Autodesk Fusion 360 part; units mm, degrees
(part 2 of 4)
sketch "Sketch14" plane through (0, 0, 0.5) normal (0, 0, 1) x (-1, 0, 0)
  circle A0 centre (101.6789, -8.3211) radius 5
  circle A1 centre (108.75, -80) radius 2
  circle A2 centre (86.25, -80) radius 2
  circle A3 centre (63.75, -80) radius 2
  circle A4 centre (41.25, -77.5) radius 2
  circle A5 centre (73.3947, -36.6053) radius 5
  circle A6 centre (87.5368, -22.4632) radius 5
  line L0 (120, -80) -> (120, 10)
  line L1 (120, 10) -> (75, 10)
  line L2 (75, 10) -> (30, 0)
  line L3 (30, 0) -> (0, 0)
  line L4 (0, 0) -> (-45, 10)
  line L5 (-45, 10) -> (-75.7574, 10)
  line L6 (-75.7574, 10) -> (-181.8234, 116.066)
  line L7 (-181.8234, 116.066) -> (-195.9655, 101.9239)
  line L8 (-195.9655, 101.9239) -> (-90, -4.0416)
  line L9 (-90, -4.0416) -> (-90, -62.2885)
  line L10 (-90, -62.2885) -> (-190, -62.2885)
  line L11 (-190, -62.2885) -> (-190, -75)
  line L12 (-190, -75) -> (-90, -75)
  line L13 (-90, -75) -> (-90, -80)
  line L14 (-90, -80) -> (-22.5, -80)
  line L15 (-22.5, -80) -> (0, -75)
  line L16 (0, -75) -> (30, -75)
  line L17 (30, -75) -> (37.3453, -76.6323)
  line L18 (37.3453, -76.6323) -> (37.3453, -83.3677)
  line L19 (37.3453, -83.3677) -> (45.1547, -83.3677)
  line L20 (45.1547, -83.3677) -> (45.1547, -78.3677)
  line L21 (45.1547, -78.3677) -> (52.5, -80)
  line L22 (52.5, -80) -> (59.75, -80)
  line L23 (59.75, -80) -> (59.75, -85)
  line L24 (59.75, -85) -> (67.75, -85)
  line L25 (67.75, -85) -> (67.75, -80)
  line L26 (67.75, -80) -> (82.25, -80)
  line L27 (82.25, -80) -> (82.25, -85)
  line L28 (82.25, -85) -> (90.25, -85)
  line L29 (90.25, -85) -> (90.25, -80)
  line L30 (90.25, -80) -> (104.75, -80)
  line L31 (104.75, -80) -> (104.75, -85)
  line L32 (104.75, -85) -> (112.75, -85)
  line L33 (112.75, -85) -> (112.75, -80)
  line L34 (112.75, -80) -> (120, -80)
  line L35 (-14.25, -68.5) -> (-8.25, -68.5)
  line L36 (-8.25, -68.5) -> (-8.25, -71.5)
  line L37 (-8.25, -71.5) -> (-14.25, -71.5)
  line L38 (-14.25, -71.5) -> (-14.25, -68.5)
  line L39 (-72.1594, -47.0213) -> (-67.271, -50.5004)
  line L40 (-67.271, -50.5004) -> (-69.0348, -52.9787)
  line L41 (-69.0348, -52.9787) -> (-73.9232, -49.4996)
  line L42 (-73.9232, -49.4996) -> (-72.1594, -47.0213)
  line L43 (-58.1594, -27.0213) -> (-53.271, -30.5004)
  line L44 (-53.271, -30.5004) -> (-55.0348, -32.9787)
  line L45 (-55.0348, -32.9787) -> (-59.9232, -29.4996)
  line L46 (-59.9232, -29.4996) -> (-58.1594, -27.0213)
  line L47 (-10.5728, -3.1023) -> (-4.573, -3.1532)
  line L48 (-4.573, -3.1532) -> (-4.5984, -6.1531)
  line L49 (-4.5984, -6.1531) -> (-10.5982, -6.1022)
  line L50 (-10.5982, -6.1022) -> (-10.5728, -3.1023)
  line L51 (-67.8203, 7.9003) -> (-65.8203, 7.9003)
  line L52 (-65.8203, 7.9003) -> (-65.8203, 5.9003)
  line L53 (-65.8203, 5.9003) -> (-67.8203, 5.9003)
  line L54 (-67.8203, 5.9003) -> (-67.8203, 7.9003)
  line L55 (-76.9306, -16.181) -> (-75.5164, -17.5952)
  line L56 (-75.5164, -17.5952) -> (-76.9306, -19.0095)
  line L57 (-76.9306, -19.0095) -> (-78.3448, -17.5952)
  line L58 (-78.3448, -17.5952) -> (-76.9306, -16.181)
  line L59 (-87.8309, -27.9541) -> (-85.8309, -27.9541)
  line L60 (-85.8309, -27.9541) -> (-85.8309, -29.9541)
  line L61 (-85.8309, -29.9541) -> (-87.8309, -29.9541)
  line L62 (-87.8309, -29.9541) -> (-87.8309, -27.9541)
  line L63 (-66.3319, -10.7541) -> (-65.4866, -8.9415)
  line L64 (-65.4866, -8.9415) -> (-63.674, -9.7867)
  line L65 (-63.674, -9.7867) -> (-64.5193, -11.5994)
  line L66 (-64.5193, -11.5994) -> (-66.3319, -10.7541)
  line L67 (-42.179, 1.1199) -> (-36.1792, 1.0739)
  line L68 (-36.1792, 1.0739) -> (-36.2025, -1.9678)
  line L69 (-36.2025, -1.9678) -> (-42.2023, -1.9219)
  line L70 (-42.2023, -1.9219) -> (-42.179, 1.1199)
  line L71 (-10.5728, -25.1023) -> (-4.573, -25.1532)
  line L72 (-4.573, -25.1532) -> (-4.5984, -28.1531)
  line L73 (-4.5984, -28.1531) -> (-10.5982, -28.1022)
  line L74 (-10.5982, -28.1022) -> (-10.5728, -25.1023)
  line L75 (-11.9719, -47.9791) -> (-6.0721, -49.071)
  line L76 (-6.0721, -49.071) -> (-6.6181, -52.0209)
  line L77 (-6.6181, -52.0209) -> (-12.5179, -50.929)
  line L78 (-12.5179, -50.929) -> (-11.9719, -47.9791)
  line L79 (-81.75, -71.5367) -> (-75.75, -71.5367)
  line L80 (-75.75, -71.5367) -> (-75.75, -74.5367)
  line L81 (-75.75, -74.5367) -> (-81.75, -74.5367)
  line L82 (-81.75, -74.5367) -> (-81.75, -71.5367)
  line L83 (-36.75, -71.5367) -> (-30.75, -71.5367)
  line L84 (-30.75, -71.5367) -> (-30.75, -74.5367)
  line L85 (-30.75, -74.5367) -> (-36.75, -74.5367)
  line L86 (-36.75, -74.5367) -> (-36.75, -71.5367)
  line L87 (-50.7607, -47.5524) -> (-45.1333, -49.6339)
  line L88 (-45.1333, -49.6339) -> (-46.174, -52.4476)
  line L89 (-46.174, -52.4476) -> (-51.8014, -50.3661)
  line L90 (-51.8014, -50.3661) -> (-50.7607, -47.5524)
  line L91 (-43.7607, -25.5524) -> (-38.1333, -27.6339)
  line L92 (-38.1333, -27.6339) -> (-39.174, -30.4476)
  line L93 (-39.174, -30.4476) -> (-44.8014, -28.3661)
  line L94 (-44.8014, -28.3661) -> (-43.7607, -25.5524)
  line L95 (-24.686, 0.859) -> (-18.6861, 0.8794)
  line L96 (-18.6861, 0.8794) -> (-18.6759, -2.1206)
  line L97 (-18.6759, -2.1206) -> (-24.6759, -2.141)
  line L98 (-24.6759, -2.141) -> (-24.686, 0.859)
  line L99 (-62.1634, 5.9003) -> (-62.1634, 7.9003)
  line L100 (-62.1634, 7.9003) -> (-60.1634, 7.9003)
  line L101 (-60.1634, 7.9003) -> (-60.1634, 5.9003)
  line L102 (-60.1634, 5.9003) -> (-62.1634, 5.9003)
  line L103 (-72.9306, -20.181) -> (-71.5164, -21.5952)
  line L104 (-71.5164, -21.5952) -> (-72.9306, -23.0095)
  line L105 (-72.9306, -23.0095) -> (-74.3448, -21.5952)
  line L106 (-74.3448, -21.5952) -> (-72.9306, -20.181)
  line L107 (-87.8309, -19.8881) -> (-85.8309, -19.8881)
  line L108 (-85.8309, -19.8881) -> (-85.8309, -21.8881)
  line L109 (-85.8309, -21.8881) -> (-87.8309, -21.8881)
  line L110 (-87.8309, -21.8881) -> (-87.8309, -19.8881)
  line L111 (-70.6135, -6.5508) -> (-68.8009, -7.396)
  line L112 (-68.8009, -7.396) -> (-69.6461, -9.2087)
  line L113 (-69.6461, -9.2087) -> (-71.4587, -8.3634)
  line L114 (-71.4587, -8.3634) -> (-70.6135, -6.5508)
  line L115 (-35.0324, 0.9507) -> (-29.0325, 0.9195)
  line L116 (-29.0325, 0.9195) -> (-29.0481, -2.0804)
  line L117 (-29.0481, -2.0804) -> (-35.048, -2.0492)
  line L118 (-35.048, -2.0492) -> (-35.0324, 0.9507)
  line L119 (-28.0908, -25.011) -> (-22.1784, -26.0328)
  line L120 (-22.1784, -26.0328) -> (-22.6893, -28.989)
  line L121 (-22.6893, -28.989) -> (-28.6017, -27.9672)
  line L122 (-28.6017, -27.9672) -> (-28.0908, -25.011)
  line L123 (-26.6893, -51.989) -> (-32.6017, -50.9672)
  line L124 (-32.6017, -50.9672) -> (-32.0908, -48.011)
  line L125 (-32.0908, -48.011) -> (-26.1784, -49.0328)
  line L126 (-26.1784, -49.0328) -> (-26.6893, -51.989)
  line L127 (-59.25, -71.5367) -> (-53.25, -71.5367)
  line L128 (-53.25, -71.5367) -> (-53.25, -74.5367)
  line L129 (-53.25, -74.5367) -> (-59.25, -74.5367)
  line L130 (-59.25, -74.5367) -> (-59.25, -71.5367)
  line L131 (-45, -57) -> (-5, -57)
  line L132 (-5, -57) -> (-5, -60)
  line L133 (-5, -60) -> (-45, -60)
  arc A7 (-45, -60) -> (-66.3234, -75) centre (-45, -82.6562) ccw
  line L134 (-66.3234, -75) -> (-69.4872, -75)
  arc A8 (-45, -57) -> (-69.4872, -75) centre (-45, -82.6562) ccw
  line L135 (0, -5) -> (30, -5)
  line L136 (30, -5) -> (30, -70)
  line L137 (30, -70) -> (0, -70)
  line L138 (0, -70) -> (0, -5)
  circle A9 centre (-167.6812, 87.7817) radius 5
  circle A10 centre (-120, -68.6442) radius 5
  circle A11 centre (-140, -68.6442) radius 5
  circle A12 centre (-153.5391, 73.6396) radius 5
  arc A13 (-87.8309, -44.505) -> (-40.6089, 7.444) centre (-128.4491, 39.8542) ccw
  line L139 (-87.8309, -44.505) -> (-87.8309, -38.9188)
  arc A14 (-87.8309, -38.9188) -> (-45.6219, 8.3158) centre (-128.4491, 39.8542) ccw
  line L140 (-45.6219, 8.3158) -> (-40.6089, 7.444)
  circle A15 centre (-181.8234, 101.9239) radius 5
  circle A16 centre (-160, -68.6442) radius 5
  circle A17 centre (-180, -68.6442) radius 5
  circle A18 centre (-139.397, 59.4975) radius 5
  circle A19 centre (-125.2548, 45.3553) radius 5
  circle A20 centre (-111.1127, 31.2132) radius 5
  line L141 (30, -70) -> (120, -70)
  line L142 (108.75, -85) -> (108.75, -59.5533)
  circle A21 centre (108.75, -70) radius 2
  circle A22 centre (105.25, -70) radius 1.5 construction
  circle A23 centre (101.75, -70) radius 2
  circle A24 centre (98.25, -70) radius 1.5 construction
  circle A25 centre (94.75, -70) radius 2
  circle A26 centre (91.25, -70) radius 1.5 construction
  circle A27 centre (87.75, -70) radius 2
  circle A28 centre (84.25, -70) radius 1.5 construction
  circle A29 centre (80.75, -70) radius 2
  circle A30 centre (77.25, -70) radius 1.5 construction
  circle A31 centre (73.75, -70) radius 2
  circle A32 centre (108.75, -70) radius 3
  circle A33 centre (101.75, -70) radius 3
  circle A34 centre (94.75, -70) radius 3
  circle A35 centre (87.75, -70) radius 3
  circle A36 centre (80.75, -70) radius 3
  circle A37 centre (73.75, -70) radius 3
  circle A38 centre (-120, -68.6442) radius 5
  circle A39 centre (-140, -68.6442) radius 5
  circle A40 centre (-160, -68.6442) radius 5
  circle A41 centre (-180, -68.6442) radius 5
  circle A42 centre (70.25, -70) radius 1.5 construction
  circle A43 centre (66.75, -70) radius 2
  circle A44 centre (63.25, -70) radius 1.5 construction
  circle A45 centre (59.75, -70) radius 2
  circle A46 centre (56.25, -70) radius 1.5 construction
  circle A47 centre (52.75, -70) radius 2
  circle A48 centre (49.25, -70) radius 1.5 construction
  circle A49 centre (45.75, -70) radius 2
  circle A50 centre (42.25, -70) radius 1.5 construction
  circle A51 centre (38.75, -70) radius 2
  circle A52 centre (66.75, -70) radius 3
  circle A53 centre (59.75, -70) radius 3
  circle A54 centre (52.75, -70) radius 3
  circle A55 centre (45.75, -70) radius 3
  circle A56 centre (38.75, -70) radius 3
  dimension "d401" = 4
  dimension "d402" = 3
  dimension "d403" = 4
  dimension "d404" = 3
  dimension "d405" = 4
  dimension "d406" = 3
  dimension "d407" = 4
  dimension "d408" = 3
  dimension "d409" = 4
  dimension "d410" = 3
  dimension "d411" = 4
  dimension "d420" = 1
  dimension "d421" = 1
  dimension "d422" = 1
  dimension "d423" = 1
  dimension "d424" = 1
  dimension "d425" = 1
  dimension "d546" = 3
  dimension "d547" = 4
  dimension "d548" = 3
  dimension "d549" = 4
  dimension "d550" = 3
  dimension "d551" = 4
  dimension "d552" = 3
  dimension "d553" = 4
  dimension "d554" = 3
  dimension "d555" = 4
  dimension "d556" = 1
  dimension "d557" = 1
  dimension "d558" = 1
  dimension "d559" = 1
  dimension "d560" = 1
  constraint coincident L136.end L137.start
  constraint coincident L0 L141.end
  constraint perpendicular L0 L141
  constraint midpoint L32 L142.start
  constraint perpendicular L141 L142
  constraint coincident L141 A21.centre
  constraint coincident L142 A21.centre
  constraint concentric A10 A38
  constraint concentric A11 A39
  constraint concentric A16 A40
  constraint concentric A17 A41
  measures "d401" diameter of A21
  measures "d402" diameter of A22
  measures "d403" diameter of A23
  measures "d404" diameter of A24
  measures "d405" diameter of A25
  measures "d406" diameter of A26
  measures "d407" diameter of A27
  measures "d408" diameter of A28
  measures "d409" diameter of A29
  measures "d410" diameter of A30
  measures "d411" diameter of A31
  measures "d546" diameter of A42
  measures "d547" diameter of A43
  measures "d548" diameter of A44
  measures "d549" diameter of A45
  measures "d550" diameter of A46
  measures "d551" diameter of A47
  measures "d552" diameter of A48
  measures "d553" diameter of A49
  measures "d554" diameter of A50
  measures "d555" diameter of A51
extrude "Extrude15" add sketch "Sketch14" along normal blind 2 contours L141 L142 A21 | L141 L142 A21 | L141 L142 A21 | L141 L142 A21 | L141 A31 | L141 A31 | L141 A29 | L141 A29 | L141 A27 | L141 A27 | L141 A25 | L141 A25 | L141 A23 | L141 A23 bodies 1
sphere "SpherePrimitive11" add diameter 5 placed x (-1, 0, 0) y (0, -1, 0) z (0, 0, 1) at (-108.75, 70, 2.5) bodies 1
sphere "SpherePrimitive12" add diameter 5 placed x (-1, 0, 0) y (0, -1, 0) z (0, 0, 1) at (-101.75, 70, 2.5) bodies 1
sphere "SpherePrimitive13" add diameter 5 placed x (-1, 0, 0) y (0, -1, 0) z (0, 0, 1) at (-94.75, 70, 2.5) bodies 1
sphere "SpherePrimitive14" add diameter 5 placed x (-1, 0, 0) y (0, -1, 0) z (0, 0, 1) at (-87.75, 70, 2.5) bodies 1
sphere "SpherePrimitive15" add diameter 5 placed x (-1, 0, 0) y (0, -1, 0) z (0, 0, 1) at (-80.75, 70, 2.5) bodies 1
sphere "SpherePrimitive16" add diameter 5 placed x (-1, 0, 0) y (0, -1, 0) z (0, 0, 1) at (-73.75, 70, 2.5) bodies 1
extrude "Extrude16" cut sketch "Sketch14" along normal blind 2 contours L141 L142 A21 A32 | L141 L142 A21 A32 | L141 L142 A21 A32 | L141 L142 A21 A32 | L141 A31 A37 | L141 A31 A37 | L141 A29 A36 | L141 A29 A36 | L141 A27 A35 | L141 A27 A35 | L141 A25 A34 | L141 A25 A34 | L141 A23 A33 | L141 A23 A33 bodies 1
extrude "Extrude17" add sketch "Sketch14" against normal blind 0.5 contours A10 A38 | A11 A39 | A16 A40 | A17 A41 bodies 1
sketch "Sketch21" plane through (0, 0, 0.5) normal (0, 0, 1) x (-1, 0, 0)
  circle A0 centre (87.75, -70) radius 2
  circle A1 centre (108.75, -70) radius 2
  circle A2 centre (80.75, -70) radius 2
  circle A3 centre (94.75, -70) radius 2
  circle A4 centre (101.75, -70) radius 2
  circle A5 centre (73.75, -70) radius 2
  circle A6 centre (101.6789, -8.3211) radius 5
  circle A7 centre (108.75, -80) radius 2
  circle A8 centre (86.25, -80) radius 2
  circle A9 centre (63.75, -80) radius 2
  circle A10 centre (41.25, -77.5) radius 2
  circle A11 centre (73.3947, -36.6053) radius 5
  circle A12 centre (87.5368, -22.4632) radius 5
  line L0 (120, -80) -> (120, 10)
  line L1 (120, 10) -> (75, 10)
  line L2 (75, 10) -> (30, 0)
  line L3 (30, 0) -> (0, 0)
  line L4 (0, 0) -> (-45, 10)
  line L5 (-45, 10) -> (-75.7574, 10)
  line L6 (-75.7574, 10) -> (-181.8234, 116.066)
  line L7 (-181.8234, 116.066) -> (-195.9655, 101.9239)
  line L8 (-195.9655, 101.9239) -> (-90, -4.0416)
  line L9 (-90, -4.0416) -> (-90, -62.2885)
  line L10 (-90, -62.2885) -> (-190, -62.2885)
  line L11 (-190, -62.2885) -> (-190, -75)
  line L12 (-190, -75) -> (-90, -75)
  line L13 (-90, -75) -> (-90, -80)
  line L14 (-90, -80) -> (-22.5, -80)
  line L15 (-22.5, -80) -> (0, -75)
  line L16 (0, -75) -> (30, -75)
  line L17 (30, -75) -> (37.3453, -76.6323)
  line L18 (37.3453, -76.6323) -> (37.3453, -83.3677)
  line L19 (37.3453, -83.3677) -> (45.1547, -83.3677)
  line L20 (45.1547, -83.3677) -> (45.1547, -78.3677)
  line L21 (45.1547, -78.3677) -> (52.5, -80)
  line L22 (52.5, -80) -> (59.75, -80)
  line L23 (59.75, -80) -> (59.75, -85)
  line L24 (59.75, -85) -> (67.75, -85)
  line L25 (67.75, -85) -> (67.75, -80)
  line L26 (67.75, -80) -> (82.25, -80)
  line L27 (82.25, -80) -> (82.25, -85)
  line L28 (82.25, -85) -> (90.25, -85)
  line L29 (90.25, -85) -> (90.25, -80)
  line L30 (90.25, -80) -> (104.75, -80)
  line L31 (104.75, -80) -> (104.75, -85)
  line L32 (104.75, -85) -> (112.75, -85)
  line L33 (112.75, -85) -> (112.75, -80)
  line L34 (112.75, -80) -> (120, -80)
  line L35 (-14.25, -68.5) -> (-8.25, -68.5)
  line L36 (-8.25, -68.5) -> (-8.25, -71.5)
  line L37 (-8.25, -71.5) -> (-14.25, -71.5)
  line L38 (-14.25, -71.5) -> (-14.25, -68.5)
  line L39 (-72.1594, -47.0213) -> (-67.271, -50.5004)
  line L40 (-67.271, -50.5004) -> (-69.0348, -52.9787)
  line L41 (-69.0348, -52.9787) -> (-73.9232, -49.4996)
  line L42 (-73.9232, -49.4996) -> (-72.1594, -47.0213)
  line L43 (-58.1594, -27.0213) -> (-53.271, -30.5004)
  line L44 (-53.271, -30.5004) -> (-55.0348, -32.9787)
  line L45 (-55.0348, -32.9787) -> (-59.9232, -29.4996)
  line L46 (-59.9232, -29.4996) -> (-58.1594, -27.0213)
  line L47 (-10.5728, -3.1023) -> (-4.573, -3.1532)
  line L48 (-4.573, -3.1532) -> (-4.5984, -6.1531)
  line L49 (-4.5984, -6.1531) -> (-10.5982, -6.1022)
  line L50 (-10.5982, -6.1022) -> (-10.5728, -3.1023)
  line L51 (-67.8203, 7.9003) -> (-65.8203, 7.9003)
  line L52 (-65.8203, 7.9003) -> (-65.8203, 5.9003)
  line L53 (-65.8203, 5.9003) -> (-67.8203, 5.9003)
  line L54 (-67.8203, 5.9003) -> (-67.8203, 7.9003)
  line L55 (-76.9306, -16.181) -> (-75.5164, -17.5952)
  line L56 (-75.5164, -17.5952) -> (-76.9306, -19.0095)
  line L57 (-76.9306, -19.0095) -> (-78.3448, -17.5952)
  line L58 (-78.3448, -17.5952) -> (-76.9306, -16.181)
  line L59 (-87.8309, -27.9541) -> (-85.8309, -27.9541)
  line L60 (-85.8309, -27.9541) -> (-85.8309, -29.9541)
  line L61 (-85.8309, -29.9541) -> (-87.8309, -29.9541)
  line L62 (-87.8309, -29.9541) -> (-87.8309, -27.9541)
  line L63 (-66.3319, -10.7541) -> (-65.4866, -8.9415)
  line L64 (-65.4866, -8.9415) -> (-63.674, -9.7867)
  line L65 (-63.674, -9.7867) -> (-64.5193, -11.5994)
  line L66 (-64.5193, -11.5994) -> (-66.3319, -10.7541)
  line L67 (-42.179, 1.1199) -> (-36.1792, 1.0739)
  line L68 (-36.1792, 1.0739) -> (-36.2025, -1.9678)
  line L69 (-36.2025, -1.9678) -> (-42.2023, -1.9219)
  line L70 (-42.2023, -1.9219) -> (-42.179, 1.1199)
  line L71 (-10.5728, -25.1023) -> (-4.573, -25.1532)
  line L72 (-4.573, -25.1532) -> (-4.5984, -28.1531)
  line L73 (-4.5984, -28.1531) -> (-10.5982, -28.1022)
  line L74 (-10.5982, -28.1022) -> (-10.5728, -25.1023)
  line L75 (-11.9719, -47.9791) -> (-6.0721, -49.071)
  line L76 (-6.0721, -49.071) -> (-6.6181, -52.0209)
  line L77 (-6.6181, -52.0209) -> (-12.5179, -50.929)
  line L78 (-12.5179, -50.929) -> (-11.9719, -47.9791)
  line L79 (-81.75, -71.5367) -> (-75.75, -71.5367)
  line L80 (-75.75, -71.5367) -> (-75.75, -74.5367)
  line L81 (-75.75, -74.5367) -> (-81.75, -74.5367)
  line L82 (-81.75, -74.5367) -> (-81.75, -71.5367)
  line L83 (-36.75, -71.5367) -> (-30.75, -71.5367)
  line L84 (-30.75, -71.5367) -> (-30.75, -74.5367)
  line L85 (-30.75, -74.5367) -> (-36.75, -74.5367)
  line L86 (-36.75, -74.5367) -> (-36.75, -71.5367)
  line L87 (-50.7607, -47.5524) -> (-45.1333, -49.6339)
  line L88 (-45.1333, -49.6339) -> (-46.174, -52.4476)
  line L89 (-46.174, -52.4476) -> (-51.8014, -50.3661)
  line L90 (-51.8014, -50.3661) -> (-50.7607, -47.5524)
  line L91 (-43.7607, -25.5524) -> (-38.1333, -27.6339)
  line L92 (-38.1333, -27.6339) -> (-39.174, -30.4476)
  line L93 (-39.174, -30.4476) -> (-44.8014, -28.3661)
  line L94 (-44.8014, -28.3661) -> (-43.7607, -25.5524)
  line L95 (-24.686, 0.859) -> (-18.6861, 0.8794)
  line L96 (-18.6861, 0.8794) -> (-18.6759, -2.1206)
  line L97 (-18.6759, -2.1206) -> (-24.6759, -2.141)
  line L98 (-24.6759, -2.141) -> (-24.686, 0.859)
  line L99 (-62.1634, 5.9003) -> (-62.1634, 7.9003)
  line L100 (-62.1634, 7.9003) -> (-60.1634, 7.9003)
  line L101 (-60.1634, 7.9003) -> (-60.1634, 5.9003)
  line L102 (-60.1634, 5.9003) -> (-62.1634, 5.9003)
  line L103 (-72.9306, -20.181) -> (-71.5164, -21.5952)
  line L104 (-71.5164, -21.5952) -> (-72.9306, -23.0095)
  line L105 (-72.9306, -23.0095) -> (-74.3448, -21.5952)
  line L106 (-74.3448, -21.5952) -> (-72.9306, -20.181)
  line L107 (-87.8309, -19.8881) -> (-85.8309, -19.8881)
  line L108 (-85.8309, -19.8881) -> (-85.8309, -21.8881)
  line L109 (-85.8309, -21.8881) -> (-87.8309, -21.8881)
  line L110 (-87.8309, -21.8881) -> (-87.8309, -19.8881)
  line L111 (-70.6135, -6.5508) -> (-68.8009, -7.396)
  line L112 (-68.8009, -7.396) -> (-69.6461, -9.2087)
  line L113 (-69.6461, -9.2087) -> (-71.4587, -8.3634)
  line L114 (-71.4587, -8.3634) -> (-70.6135, -6.5508)
  line L115 (-35.0324, 0.9507) -> (-29.0325, 0.9195)
  line L116 (-29.0325, 0.9195) -> (-29.0481, -2.0804)
  line L117 (-29.0481, -2.0804) -> (-35.048, -2.0492)
  line L118 (-35.048, -2.0492) -> (-35.0324, 0.9507)
  line L119 (-28.0908, -25.011) -> (-22.1784, -26.0328)
  line L120 (-22.1784, -26.0328) -> (-22.6893, -28.989)
  line L121 (-22.6893, -28.989) -> (-28.6017, -27.9672)
  line L122 (-28.6017, -27.9672) -> (-28.0908, -25.011)
  line L123 (-26.6893, -51.989) -> (-32.6017, -50.9672)
  line L124 (-32.6017, -50.9672) -> (-32.0908, -48.011)
  line L125 (-32.0908, -48.011) -> (-26.1784, -49.0328)
  line L126 (-26.1784, -49.0328) -> (-26.6893, -51.989)
  line L127 (-59.25, -71.5367) -> (-53.25, -71.5367)
  line L128 (-53.25, -71.5367) -> (-53.25, -74.5367)
  line L129 (-53.25, -74.5367) -> (-59.25, -74.5367)
  line L130 (-59.25, -74.5367) -> (-59.25, -71.5367)
  line L131 (-45, -57) -> (-5, -57)
  line L132 (-5, -57) -> (-5, -60)
  line L133 (-5, -60) -> (-45, -60)
  arc A13 (-45, -60) -> (-66.3234, -75) centre (-45, -82.6562) ccw
  line L134 (-66.3234, -75) -> (-69.4872, -75)
  arc A14 (-45, -57) -> (-69.4872, -75) centre (-45, -82.6562) ccw
  line L135 (0, -5) -> (30, -5)
  line L136 (30, -5) -> (30, -70)
  line L137 (30, -70) -> (0, -70)
  line L138 (0, -70) -> (0, -5)
  circle A15 centre (-167.6812, 87.7817) radius 5
  circle A16 centre (-153.5391, 73.6396) radius 5
  arc A17 (-87.8309, -44.505) -> (-40.6089, 7.444) centre (-128.4491, 39.8542) ccw
  line L139 (-87.8309, -44.505) -> (-87.8309, -38.9188)
  arc A18 (-87.8309, -38.9188) -> (-45.6219, 8.3158) centre (-128.4491, 39.8542) ccw
  line L140 (-45.6219, 8.3158) -> (-40.6089, 7.444)
  circle A19 centre (-181.8234, 101.9239) radius 5
  circle A20 centre (-139.397, 59.4975) radius 5
  circle A21 centre (-125.2548, 45.3553) radius 5
  circle A22 centre (-111.1127, 31.2132) radius 5
  line L141 (-190, -68.6442) -> (-89.9719, -68.6442) construction
  circle A23 centre (-187.5, -68.6442) radius 2.5 construction
  circle A24 centre (-183, -68.6442) radius 2
  circle A25 centre (-179.5, -68.6442) radius 1.5 construction
  circle A26 centre (-176, -68.6442) radius 2
  circle A27 centre (-172.5, -68.6442) radius 1.5 construction
  circle A28 centre (-169, -68.6442) radius 2
  circle A29 centre (-165.5, -68.6442) radius 1.5 construction
  circle A30 centre (-162, -68.6442) radius 2
  circle A31 centre (-158.5, -68.6442) radius 1.5 construction
  circle A32 centre (-155, -68.6442) radius 2
  circle A33 centre (-151.5, -68.6442) radius 1.5 construction
  circle A34 centre (-148, -68.6442) radius 2
  circle A35 centre (-144.5, -68.6442) radius 1.5 construction
  circle A36 centre (-141, -68.6442) radius 2
  circle A37 centre (-137.5, -68.6442) radius 1.5 construction
  circle A38 centre (-134, -68.6442) radius 2
  circle A39 centre (-130.5, -68.6442) radius 1.5 construction
  circle A40 centre (-127, -68.6442) radius 2
  circle A41 centre (-123.5, -68.6442) radius 1.5 construction
  circle A42 centre (-120, -68.6442) radius 2
  circle A43 centre (-116.5, -68.6442) radius 1.5 construction
  circle A44 centre (-113, -68.6442) radius 2
  circle A45 centre (-113, -68.6442) radius 1.5
  circle A46 centre (-120, -68.6442) radius 1.5
  circle A47 centre (-127, -68.6442) radius 1.5
  circle A48 centre (-134, -68.6442) radius 1.5
  circle A49 centre (-141, -68.6442) radius 1.5
  circle A50 centre (-148, -68.6442) radius 1.5
  circle A51 centre (-155, -68.6442) radius 1.5
  circle A52 centre (-162, -68.6442) radius 1.5
  circle A53 centre (-169, -68.6442) radius 1.5
  circle A54 centre (-176, -68.6442) radius 1.5
  circle A55 centre (-183, -68.6442) radius 1.5
  circle A56 centre (-109.5, -68.6442) radius 1.5 construction
  circle A57 centre (-106, -68.6442) radius 2 construction
  circle A58 centre (-102.5, -68.6442) radius 1.5 construction
  circle A59 centre (-99, -68.6442) radius 2 construction
  circle A60 centre (-95.5, -68.6442) radius 1.5 construction
  circle A61 centre (-92, -68.6442) radius 2 construction
  circle A62 centre (-106, -68.6442) radius 1.5
  circle A63 centre (-99, -68.6442) radius 1.5
  circle A64 centre (-92, -68.6442) radius 1.5
  dimension "d430" = 5
  dimension "d431" = 4
  dimension "d432" = 3
  dimension "d433" = 4
  dimension "d434" = 3
  dimension "d435" = 4
  dimension "d436" = 3
  dimension "d437" = 4
  dimension "d438" = 3
  dimension "d439" = 4
  dimension "d440" = 3
  dimension "d441" = 4
  dimension "d442" = 3
  dimension "d443" = 4
  dimension "d444" = 3
  dimension "d445" = 4
  dimension "d446" = 3
  dimension "d447" = 4
  dimension "d448" = 3
  dimension "d449" = 4
  dimension "d450" = 3
  dimension "d451" = 4
  dimension "d454" = 3
  dimension "d455" = 3
  dimension "d456" = 3
  dimension "d457" = 3
  dimension "d458" = 3
  dimension "d459" = 3
  dimension "d460" = 3
  dimension "d461" = 3
  dimension "d462" = 3
  dimension "d463" = 3
  dimension "d464" = 3
  dimension "d530" = 3
  dimension "d531" = 4
  dimension "d532" = 3
  dimension "d533" = 4
  dimension "d534" = 3
  dimension "d535" = 4
  dimension "d536" = 3
  dimension "d537" = 3
  dimension "d538" = 3
  constraint midpoint L11 L141.start
  constraint perpendicular L11 L141
  constraint coincident L141.start A23
  constraint concentric A44 A45
  constraint concentric A42 A46
  constraint concentric A40 A47
  constraint concentric A38 A48
  constraint concentric A36 A49
  constraint concentric A34 A50
  constraint concentric A32 A51
  constraint concentric A30 A52
  constraint concentric A28 A53
  constraint concentric A26 A54
  constraint concentric A24 A55
  constraint concentric A57 A62
  constraint concentric A59 A63
  constraint concentric A61 A64
  measures "d430" diameter of A23
  measures "d431" diameter of A24
  measures "d432" diameter of A25
  measures "d433" diameter of A26
  measures "d434" diameter of A27
  measures "d435" diameter of A28
  measures "d436" diameter of A29
  measures "d437" diameter of A30
  measures "d438" diameter of A31
  measures "d439" diameter of A32
  measures "d440" diameter of A33
  measures "d441" diameter of A34
  measures "d442" diameter of A35
  measures "d443" diameter of A36
  measures "d444" diameter of A37
  measures "d445" diameter of A38
  measures "d446" diameter of A39
  measures "d447" diameter of A40
  measures "d448" diameter of A41
  measures "d449" diameter of A42
  measures "d450" diameter of A43
  measures "d451" diameter of A44
  measures "d454" diameter of A45
  measures "d455" diameter of A46
  measures "d456" diameter of A47
  measures "d457" diameter of A48
  measures "d458" diameter of A49
  measures "d459" diameter of A50
  measures "d460" diameter of A51
  measures "d461" diameter of A52
  measures "d462" diameter of A53
  measures "d463" diameter of A54
  measures "d464" diameter of A55
  measures "d530" diameter of A56
  measures "d531" diameter of A57
  measures "d532" diameter of A58
  measures "d533" diameter of A59
  measures "d534" diameter of A60
  measures "d535" diameter of A61
  measures "d536" diameter of A62
  measures "d537" diameter of A63
  measures "d538" diameter of A64
extrude "Extrude18" cut sketch "Sketch21" against normal blind 3 contours A24 | A26 | A28 | A30 | A32 | A34 | A36 | A38 | A40 | A42 | A44 | A45 | A46 | A47 | A48 | A49 | A50 | A51 | A52 | A53 | A54 | A55 bodies 1
extrude "Extrude19" add sketch "Sketch1" along normal blind 0.5 contours A5 | A7 | A9 | A11 | A13 | A15 bodies 1
extrude "Extrude20" add sketch "Sketch21" against normal blind 0.5 contours A24 | A26 | A28 | A30 | A32 | A34 | A36 | A38 | A40 | A42 | A44 bodies 1
extrude "Extrude21" add 16 faces at (79.75, 72.5367, 2) (57.25, 72.5367, 2) (32.75, 72.5367, 2) (12.25, 69.5, 2) (30.4606, 50.3224, 2) (47.7029, 50.8159, 2) (71.1179, 49.0071, 2) (57.7058, 29.8332, 2) (40.7029, 28.8159, 2) (24.4898, 27.663, 2) (8.4027, 50.6736, 2) (8.5898, 27.1192, 2) (8.5898, 5.1192, 2) (22.6793, 1.1342, 2) (33.0428, 1.0596, 2) (40.1868, -0.0907, 2) along direction (0, 0, 1) blind 4 on bodies 1 bodies 1
hole "Hole57" at (56.25, 74.5367, 3.25) direction (0, -1, 0) diameter 2 depth 5 tip angle 118 bodies 1
hole "Hole58" at (78.75, 74.5367, 3.25) direction (0, -1, 0) diameter 2 depth 5 tip angle 118 bodies 1
hole "Hole59" at (71.479, 51.2392, 3.25) direction (-0.579837, -0.814733, 0) diameter 1.6 depth 5 tip angle 118 bodies 1
hole "Hole60" at (57.479, 31.2392, 3.25) direction (-0.579837, -0.814733, 0) diameter 1.6 depth 5 tip angle 118 bodies 1
hole "Hole61" at (39.2024, 1.9449, 3.25) direction (-0.007663, -0.999971, 0) diameter 1.7 depth 5 tip angle 118 bodies 1
hole "Hole62" at (32.048, 2.0648, 3.25) direction (-0.005199, -0.999986, 0) diameter 1.7 depth 5 tip angle 118 bodies 1
hole "Hole63" at (21.6759, 2.1308, 3.25) direction (0.003391, -0.999994, 0) diameter 1.7 depth 5 tip angle 118 bodies 1
hole "Hole64" at (7.5983, 6.1277, 3.25) direction (-0.008481, -0.999964, 0) diameter 1.7 depth 5 tip angle 118 bodies 1
hole "Hole65" at (25.6455, 28.4781, 3.25) direction (-0.170308, -0.985391, 0) diameter 1.7 depth 5 tip angle 118 bodies 1
hole "Hole66" at (41.9877, 29.4069, 3.25) direction (-0.346901, -0.937902, 0) diameter 2 depth 5 tip angle 118 bodies 1
hole "Hole67" at (48.9877, 51.4069, 3.25) direction (-0.346901, -0.937902, 0) diameter 2 depth 5 tip angle 118 bodies 1
hole "Hole68" at (29.6455, 51.4781, 3.25) direction (-0.170308, -0.985391, 0) diameter 2 depth 5 tip angle 118 bodies 1
hole "Hole69" at (33.75, 74.5367, 3.25) direction (0, -1, 0) diameter 2 depth 5 tip angle 118 bodies 1
hole "Hole70" at (11.25, 71.5, 3.25) direction (0, -1, 0) diameter 2 depth 5 tip angle 118 bodies 1
hole "Hole71" at (9.568, 51.4749, 3.25) direction (-0.181994, -0.9833, 0) diameter 2 depth 5 tip angle 118 bodies 1
hole "Hole72" at (7.5983, 28.1277, 3.25) direction (-0.008481, -0.999964, 0) diameter 2 depth 5 tip angle 118 bodies 1
sketch "Sketch22" plane through (0, 0, 0.5) normal (0, 0, 1) x (-1, 0, 0)
  circle A0 centre (-183, -68.6442) radius 1.5
  circle A1 centre (-155, -68.6442) radius 1.5
  circle A2 centre (-127, -68.6442) radius 1.5
  circle A3 centre (-120, -68.6442) radius 1.5
  circle A4 centre (-148, -68.6442) radius 1.5
  circle A5 centre (-176, -68.6442) radius 1.5
  circle A6 centre (-162, -68.6442) radius 1.5
  circle A7 centre (-134, -68.6442) radius 1.5
  circle A8 centre (-113, -68.6442) radius 1.5
  circle A9 centre (-141, -68.6442) radius 1.5
  circle A10 centre (-169, -68.6442) radius 1.5
  circle A11 centre (-181.8234, 101.9239) radius 4.5
  circle A12 centre (-125.2548, 45.3553) radius 4.5
  circle A13 centre (-139.397, 59.4975) radius 4.5
  circle A14 centre (-167.6812, 87.7817) radius 4.5
  circle A15 centre (-111.1127, 31.2132) radius 4.5
  circle A16 centre (-153.5391, 73.6396) radius 4.5
  circle A17 centre (87.75, -70) radius 2
  circle A18 centre (108.75, -70) radius 2
  circle A19 centre (80.75, -70) radius 2
  circle A20 centre (94.75, -70) radius 2
  circle A21 centre (101.75, -70) radius 2
  circle A22 centre (73.75, -70) radius 2
  circle A23 centre (101.6789, -8.3211) radius 5
  circle A24 centre (108.75, -80) radius 2
  circle A25 centre (86.25, -80) radius 2
  circle A26 centre (63.75, -80) radius 2
  circle A27 centre (41.25, -77.5) radius 2
  circle A28 centre (73.3947, -36.6053) radius 5
  circle A29 centre (87.5368, -22.4632) radius 5
  line L0 (120, -80) -> (120, 10)
  line L1 (120, 10) -> (75, 10)
  line L2 (75, 10) -> (30, 0)
  line L3 (30, 0) -> (0, 0)
  line L4 (0, 0) -> (-45, 10)
  line L5 (-45, 10) -> (-75.7574, 10)
  line L6 (-75.7574, 10) -> (-181.8234, 116.066)
  line L7 (-181.8234, 116.066) -> (-195.9655, 101.9239)
  line L8 (-195.9655, 101.9239) -> (-90, -4.0416)
  line L9 (-90, -4.0416) -> (-90, -62.2885)
  line L10 (-90, -62.2885) -> (-190, -62.2885)
  line L11 (-190, -62.2885) -> (-190, -75)
  line L12 (-190, -75) -> (-90, -75)
  line L13 (-90, -75) -> (-90, -80)
  line L14 (-90, -80) -> (-22.5, -80)
  line L15 (-22.5, -80) -> (0, -75)
  line L16 (0, -75) -> (30, -75)
  line L17 (30, -75) -> (37.3453, -76.6323)
  line L18 (37.3453, -76.6323) -> (37.3453, -83.3677)
  line L19 (37.3453, -83.3677) -> (45.1547, -83.3677)
  line L20 (45.1547, -83.3677) -> (45.1547, -78.3677)
  line L21 (45.1547, -78.3677) -> (52.5, -80)
  line L22 (52.5, -80) -> (59.75, -80)
  line L23 (59.75, -80) -> (59.75, -85)
  line L24 (59.75, -85) -> (67.75, -85)
  line L25 (67.75, -85) -> (67.75, -80)
  line L26 (67.75, -80) -> (82.25, -80)
  line L27 (82.25, -80) -> (82.25, -85)
  line L28 (82.25, -85) -> (90.25, -85)
  line L29 (90.25, -85) -> (90.25, -80)
  line L30 (90.25, -80) -> (104.75, -80)
  line L31 (104.75, -80) -> (104.75, -85)
  line L32 (104.75, -85) -> (112.75, -85)
  line L33 (112.75, -85) -> (112.75, -80)
  line L34 (112.75, -80) -> (120, -80)
  line L35 (-14.25, -68.5) -> (-8.25, -68.5)
  line L36 (-8.25, -68.5) -> (-8.25, -71.5)
  line L37 (-8.25, -71.5) -> (-14.25, -71.5)
  line L38 (-14.25, -71.5) -> (-14.25, -68.5)
  line L39 (-72.1594, -47.0213) -> (-67.271, -50.5004)
  line L40 (-67.271, -50.5004) -> (-69.0348, -52.9787)
  line L41 (-69.0348, -52.9787) -> (-73.9232, -49.4996)
  line L42 (-73.9232, -49.4996) -> (-72.1594, -47.0213)
  line L43 (-58.1594, -27.0213) -> (-53.271, -30.5004)
  line L44 (-53.271, -30.5004) -> (-55.0348, -32.9787)
  line L45 (-55.0348, -32.9787) -> (-59.9232, -29.4996)
  line L46 (-59.9232, -29.4996) -> (-58.1594, -27.0213)
  line L47 (-10.5728, -3.1023) -> (-4.573, -3.1532)
  line L48 (-4.573, -3.1532) -> (-4.5984, -6.1531)
  line L49 (-4.5984, -6.1531) -> (-10.5982, -6.1022)
  line L50 (-10.5982, -6.1022) -> (-10.5728, -3.1023)
  line L51 (-67.8203, 7.9003) -> (-65.8203, 7.9003)
  line L52 (-65.8203, 7.9003) -> (-65.8203, 5.9003)
  line L53 (-65.8203, 5.9003) -> (-67.8203, 5.9003)
  line L54 (-67.8203, 5.9003) -> (-67.8203, 7.9003)
  line L55 (-76.9306, -16.181) -> (-75.5164, -17.5952)
  line L56 (-75.5164, -17.5952) -> (-76.9306, -19.0095)
  line L57 (-76.9306, -19.0095) -> (-78.3448, -17.5952)
  line L58 (-78.3448, -17.5952) -> (-76.9306, -16.181)
  line L59 (-87.8309, -27.9541) -> (-85.8309, -27.9541)
  line L60 (-85.8309, -27.9541) -> (-85.8309, -29.9541)
  line L61 (-85.8309, -29.9541) -> (-87.8309, -29.9541)
  line L62 (-87.8309, -29.9541) -> (-87.8309, -27.9541)
  line L63 (-66.3319, -10.7541) -> (-65.4866, -8.9415)
  line L64 (-65.4866, -8.9415) -> (-63.674, -9.7867)
  line L65 (-63.674, -9.7867) -> (-64.5193, -11.5994)
  line L66 (-64.5193, -11.5994) -> (-66.3319, -10.7541)
  line L67 (-42.179, 1.1199) -> (-36.1792, 1.0739)
  line L68 (-36.1792, 1.0739) -> (-36.2025, -1.9678)
  line L69 (-36.2025, -1.9678) -> (-42.2023, -1.9219)
  line L70 (-42.2023, -1.9219) -> (-42.179, 1.1199)
  line L71 (-10.5728, -25.1023) -> (-4.573, -25.1532)
  line L72 (-4.573, -25.1532) -> (-4.5984, -28.1531)
  line L73 (-4.5984, -28.1531) -> (-10.5982, -28.1022)
  line L74 (-10.5982, -28.1022) -> (-10.5728, -25.1023)
  line L75 (-11.9719, -47.9791) -> (-6.0721, -49.071)
  line L76 (-6.0721, -49.071) -> (-6.6181, -52.0209)
  line L77 (-6.6181, -52.0209) -> (-12.5179, -50.929)
  line L78 (-12.5179, -50.929) -> (-11.9719, -47.9791)
  line L79 (-81.75, -71.5367) -> (-75.75, -71.5367)
  line L80 (-75.75, -71.5367) -> (-75.75, -74.5367)
  line L81 (-75.75, -74.5367) -> (-81.75, -74.5367)
  line L82 (-81.75, -74.5367) -> (-81.75, -71.5367)
  line L83 (-36.75, -71.5367) -> (-30.75, -71.5367)
  line L84 (-30.75, -71.5367) -> (-30.75, -74.5367)
  line L85 (-30.75, -74.5367) -> (-36.75, -74.5367)
  line L86 (-36.75, -74.5367) -> (-36.75, -71.5367)
  line L87 (-50.7607, -47.5524) -> (-45.1333, -49.6339)
  line L88 (-45.1333, -49.6339) -> (-46.174, -52.4476)
  line L89 (-46.174, -52.4476) -> (-51.8014, -50.3661)
  line L90 (-51.8014, -50.3661) -> (-50.7607, -47.5524)
  line L91 (-43.7607, -25.5524) -> (-38.1333, -27.6339)
  line L92 (-38.1333, -27.6339) -> (-39.174, -30.4476)
  line L93 (-39.174, -30.4476) -> (-44.8014, -28.3661)
  line L94 (-44.8014, -28.3661) -> (-43.7607, -25.5524)
  line L95 (-24.686, 0.859) -> (-18.6861, 0.8794)
  line L96 (-18.6861, 0.8794) -> (-18.6759, -2.1206)
  line L97 (-18.6759, -2.1206) -> (-24.6759, -2.141)
  line L98 (-24.6759, -2.141) -> (-24.686, 0.859)
  line L99 (-62.1634, 5.9003) -> (-62.1634, 7.9003)
  line L100 (-62.1634, 7.9003) -> (-60.1634, 7.9003)
  line L101 (-60.1634, 7.9003) -> (-60.1634, 5.9003)
  line L102 (-60.1634, 5.9003) -> (-62.1634, 5.9003)
  line L103 (-72.9306, -20.181) -> (-71.5164, -21.5952)
  line L104 (-71.5164, -21.5952) -> (-72.9306, -23.0095)
  line L105 (-72.9306, -23.0095) -> (-74.3448, -21.5952)
  line L106 (-74.3448, -21.5952) -> (-72.9306, -20.181)
  line L107 (-87.8309, -19.8881) -> (-85.8309, -19.8881)
  line L108 (-85.8309, -19.8881) -> (-85.8309, -21.8881)
  line L109 (-85.8309, -21.8881) -> (-87.8309, -21.8881)
  line L110 (-87.8309, -21.8881) -> (-87.8309, -19.8881)
  line L111 (-70.6135, -6.5508) -> (-68.8009, -7.396)
  line L112 (-68.8009, -7.396) -> (-69.6461, -9.2087)
  line L113 (-69.6461, -9.2087) -> (-71.4587, -8.3634)
  line L114 (-71.4587, -8.3634) -> (-70.6135, -6.5508)
  line L115 (-35.0324, 0.9507) -> (-29.0325, 0.9195)
  line L116 (-29.0325, 0.9195) -> (-29.0481, -2.0804)
  line L117 (-29.0481, -2.0804) -> (-35.048, -2.0492)
  line L118 (-35.048, -2.0492) -> (-35.0324, 0.9507)
  line L119 (-28.0908, -25.011) -> (-22.1784, -26.0328)
  line L120 (-22.1784, -26.0328) -> (-22.6893, -28.989)
  line L121 (-22.6893, -28.989) -> (-28.6017, -27.9672)
  line L122 (-28.6017, -27.9672) -> (-28.0908, -25.011)
  line L123 (-26.6893, -51.989) -> (-32.6017, -50.9672)
  line L124 (-32.6017, -50.9672) -> (-32.0908, -48.011)
  line L125 (-32.0908, -48.011) -> (-26.1784, -49.0328)
  line L126 (-26.1784, -49.0328) -> (-26.6893, -51.989)
  line L127 (-59.25, -71.5367) -> (-53.25, -71.5367)
  line L128 (-53.25, -71.5367) -> (-53.25, -74.5367)
  line L129 (-53.25, -74.5367) -> (-59.25, -74.5367)
  line L130 (-59.25, -74.5367) -> (-59.25, -71.5367)
  line L131 (-45, -57) -> (-5, -57)
  line L132 (-5, -57) -> (-5, -60)
  line L133 (-5, -60) -> (-45, -60)
  arc A30 (-45, -60) -> (-66.3234, -75) centre (-45, -82.6562) ccw
  line L134 (-66.3234, -75) -> (-69.4872, -75)
  arc A31 (-45, -57) -> (-69.4872, -75) centre (-45, -82.6562) ccw
  arc A32 (-87.8309, -44.505) -> (-40.6089, 7.444) centre (-128.4491, 39.8542) ccw
  line L135 (-87.8309, -44.505) -> (-87.8309, -38.9188)
  arc A33 (-87.8309, -38.9188) -> (-45.6219, 8.3158) centre (-128.4491, 39.8542) ccw
  line L136 (-45.6219, 8.3158) -> (-40.6089, 7.444)
  line L137 (0, -5) -> (30, -5)
  line L138 (30, -5) -> (30, -70)
  line L139 (30, -70) -> (0, -70)
  line L140 (0, -70) -> (0, -5)
  line L141 (0, -9.2623) -> (-5, -9.2623) construction
  line L142 (-5, -9.2623) -> (-5.0969, -20.6836)
  line L143 (-5.0969, -20.6836) -> (-49.2268, -20.3093)
  line L144 (-49.2268, -20.3093) -> (-41.9977, -4.5677)
  line L145 (-41.9977, -4.5677) -> (-17.7598, -4.7733)
  line L146 (-17.7598, -4.7733) -> (-5, -9.2623)
  line L147 (-64.4557, -34.7655) -> (-5, -35.2698)
  line L148 (-5, -35.2698) -> (-5.0893, -45.8041)
  line L149 (-5.0893, -45.8041) -> (-79.6826, -45.1714)
  line L150 (-79.6826, -45.1714) -> (-64.4557, -34.7655)
  line L151 (-87.8309, -48.5956) -> (-64.4557, -59.7611)
  line L152 (-64.4557, -59.7611) -> (-70.6729, -68.3891)
  line L153 (-70.6729, -68.3891) -> (-87.8309, -68.3891)
  line L154 (-87.8309, -68.3891) -> (-87.8309, -48.5956)
  line L155 (30, -5) -> (35, -5) construction
  line L156 (35, -5) -> (80, 5)
  line L157 (80, 5) -> (115, 5)
  line L158 (99.8546, 5) -> (35, -50.5455)
  line L159 (115, -15.9161) -> (115, -61.1347)
  line L160 (115, -61.1347) -> (67.4273, -61.1347)
  line L161 (67.4273, -61.1347) -> (115, -15.9161)
  line L162 (35, -5) -> (35, -50.5455)
  dimension "d525" = 5
  dimension "d526" = 5
  dimension "d527" = 35
  constraint coincident L140 L141.start
  constraint perpendicular L140 L141
  constraint perpendicular L71 L142
  constraint perpendicular L142 L143
  constraint perpendicular L142 L145
  constraint parallel L143 L147
  constraint perpendicular L147 L148
  constraint perpendicular L148 L149
  constraint perpendicular L135 L153
  constraint perpendicular L153 L154
  constraint coincident L137.end L138.start
  constraint perpendicular L0 L155
  constraint parallel L2 L156
  constraint perpendicular L0 L157
  constraint coincident L157 L158.start
  constraint perpendicular L157 L159
  constraint perpendicular L159 L160
  constraint perpendicular L155 L162
  measures "d525" distance of L141.start L141.end
  measures "d526" distance of L137.end L155.end
  measures "d527" distance of L156.end L157.end
extrude "Extrude22" cut sketch "Sketch22" against normal blind 30 contours L142 L143 L144 L145 L146 | L147 L148 L149 L150 | L151 L152 L153 L154 | L156 L157 L158 L162 | L159 L160 L161 bodies 1
extrude "Extrude23" cut sketch "Sketch1" along normal blind 4 contours A32 bodies 1
extrude "Extrude24" cut sketch "Sketch21" against normal blind 3 contours A62 | A63 | A64 bodies 1
extrude "Extrude25" add sketch "Sketch14" along normal blind 2 contours L141 A51 | L141 A51 | L141 A49 | L141 A49 | L141 A47 | L141 A47 | L141 A45 | L141 A45 | L141 A43 | L141 A43 bodies 1
sphere "SpherePrimitive17" add diameter 5 placed x (-1, 0, 0) y (0, -1, 0) z (0, 0, 1) at (-66.75, 70, 2.5) bodies 1
sphere "SpherePrimitive18" add diameter 5 placed x (-1, 0, 0) y (0, -1, 0) z (0, 0, 1) at (-59.75, 70, 2.5) bodies 1
sphere "SpherePrimitive19" add diameter 5 placed x (-1, 0, 0) y (0, -1, 0) z (0, 0, 1) at (-52.75, 70, 2.5) bodies 1
sphere "SpherePrimitive20" add diameter 5 placed x (-1, 0, 0) y (0, -1, 0) z (0, 0, 1) at (-45.75, 70, 2.5) bodies 1
sphere "SpherePrimitive21" add diameter 5 placed x (-1, 0, 0) y (0, -1, 0) z (0, 0, 1) at (-38.75, 70, 2.5) bodies 1
extrude "Extrude26" cut sketch "Sketch14" along normal blind 2 contours L141 A51 A56 | L141 A51 A56 | L141 A49 A55 | L141 A49 A55 | L141 A47 A54 | L141 A47 A54 | L141 A45 A53 | L141 A45 A53 | L141 A43 A52 | L141 A43 A52 bodies 1